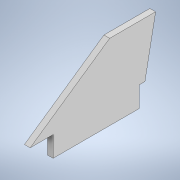
# Autodesk Inventor part: Fin
Saved by Autodesk Inventor 2022 (Build 260153000, 153)
## iProperties
Created: 2021-10-30
Part Number: Fin
Material: Generic
Document SubType Name: Modeling
Designer: Ryan
Density: 1 g/cm^3
Appearance: Default
Author: Ryan
Autodesk Inventor part; units mm, degrees
ref_plane "YZ Plane" through (0, 0, 0) normal (1, 0, 0) x (0, 1, 0)
ref_plane "XZ Plane" through (0, 0, 0) normal (0, 1, 0) x (-1, 0, 0)
ref_plane "XY Plane" through (0, 0, 0) normal (0, 0, 1) x (1, 0, 0)
sketch "Sketch1" plane through (0, 0, 0) normal (1, 0, 0) x (0, 1, 0)
  line L0 (0, 127) -> (60.96, 38.9626)
  line L1 (0, 127) -> (107.0827, 127) construction
  line L2 (60.96, 38.9626) -> (60.96, -11.8374)
  line L3 (60.96, -11.8374) -> (0, 0)
  line L4 (0, 127) -> (0, 101.6)
  line L5 (0, 101.6) -> (-22.733, 101.6)
  line L6 (-22.733, 101.6) -> (-22.733, 6.35)
  line L7 (-22.733, 6.35) -> (0, 6.35)
  line L8 (0, 0) -> (0, 6.35)
  line L9 (0, 101.6) -> (0, 127)
  dimension "d0" = 127
  dimension "d1" = 55.3
  dimension "d3" = 50.8
  dimension "d4" = 25.4
  dimension "d5" = 22.733
  dimension "d6" = 95.25
  constraints: 20 end point, 4 perpendicular, 3 vertical, 1 equal length, 1 horizontal
  measures "d0" distance of L3.end L0.start
  measures "d1" angle of L0 L1
  measures "d3" distance of L0.end L2.end
  measures "d4" distance of L0.start L4.end
  measures "d5" distance of L4.end L5.end
  measures "d6" distance of L5.end L6.end
extrude "Extrusion1" add sketch "Sketch1" along normal blind 6.35
body "Solid1"
